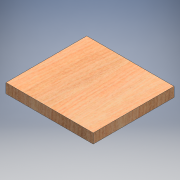
# Autodesk Inventor part: 240626_tablep1
Saved by Autodesk Inventor 2016 (Build 200138000, 138)
## iProperties
Created: 2024-06-26
Part Number: 240626_tablep1
Material: 일반
Document SubType Name: Modeling
Designer: pc
Density: 1 g/cm^3
Appearance: 자작나무 - 내츄럴 연마
Author: pc
Autodesk Inventor part; units mm, degrees
ref_plane "YZ Plane" through (0, 0, 0) normal (1, 0, 0) x (0, 1, 0)
ref_plane "XZ Plane" through (0, 0, 0) normal (0, 1, 0) x (-1, 0, 0)
ref_plane "XY Plane" through (0, 0, 0) normal (0, 0, 1) x (1, 0, 0)
sketch "스케치1" plane through (0, 0, 0) normal (0, 0, 1) x (1, 0, 0)
  line L0 (135, -125) -> (-135, -125)
  line L1 (-135, -125) -> (-135, 125)
  line L2 (-135, 125) -> (135, 125)
  line L3 (135, 125) -> (135, -125)
  line L4 (135, -125) -> (-135, 125) construction
  line L5 (-135, -125) -> (135, 125) construction
  point P0 (0, 0)
  dimension "d0" = 270
  dimension "d1" = 250
  constraints: 12 end point, 2 midpoint, 2 parallel, 1 horizontal, 1 perpendicular
  measures "d0" distance of L1.end L2.end
  measures "d1" distance of L0.end L1.end
extrude "돌출1" add sketch "스케치1" along normal blind 30
